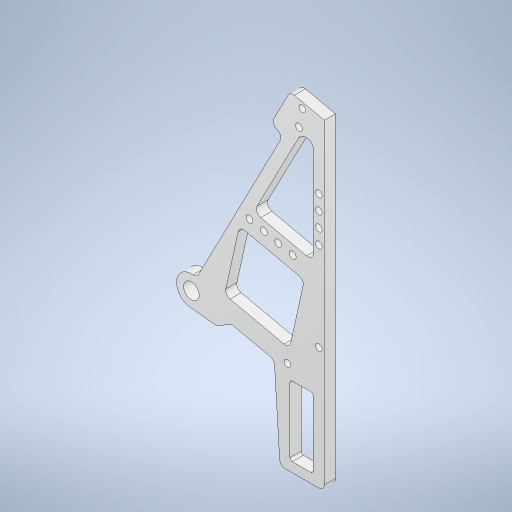
# Autodesk Inventor part: Uprights
Saved by Autodesk Inventor 2023.4 (Build 274418000, 418)
## iProperties
Created: 2024-02-11
Part Number: Uprights
Material: Aluminum 6061
Document SubType Name: Modeling
Designer: Nathan Cai
Density: 2.7 g/cm^3
Appearance: Aluminum - Flat
Mass: 24.6883 g
Surface Area: 68.1147 cm^2
Volume: 9.14381 cm^3
Author: Nathan Cai
Autodesk Inventor part; units mm, degrees
ref_plane "YZ Plane" through (0, 0, 0) normal (1, 0, 0) x (0, 1, 0)
ref_plane "XZ Plane" through (0, 0, 0) normal (0, 1, 0) x (-1, 0, 0)
ref_plane "XY Plane" through (0, 0, 0) normal (0, 0, 1) x (1, 0, 0)
sketch "Sketch1" plane through (0, 0, 0) normal (0, 0, 1) x (1, 0, 0)
  line L0 (0, 0) -> (0, 136.2362)
  line L1 (-14.9636, 12.2907) -> (-42.8613, 18.4755)
  line L2 (-42.8613, 18.4755) -> (-36.5047, 47.1481)
  line L3 (-36.5047, 47.1481) -> (-8.607, 40.9633)
  line L4 (-8.607, 40.9633) -> (-14.9636, 12.2907)
  line L5 (-42.8613, 18.4755) -> (-8.607, 40.9633) construction
  line L6 (-36.5047, 47.1481) -> (-14.9636, 12.2907) construction
  circle A0 centre (-57.15, 12.7) radius 3.3401
  circle A1 centre (-57.15, 12.7) radius 6.35
  line L7 (0, 0) -> (-57.847, 6.3884)
  line L8 (-62.7825, 15.6321) -> (0, 136.2362)
  line L9 (-30.3052, 45.7737) -> (-40.6279, 28.5497)
  line L10 (-14.8065, 42.3377) -> (-12.7302, 22.3649)
  line L11 (-22.5559, 44.0557) -> (-28.9124, 15.3831) construction
  line L12 (0, 104.775) -> (-14.6831, 108.0302)
  line L13 (-40.1014, 8.9204) -> (-21.503, 4.7972)
  line L14 (-21.503, 4.7972) -> (-22.8774, -1.4022)
  line L15 (-22.8774, -1.4022) -> (-41.4758, 2.7209)
  line L16 (-41.4758, 2.7209) -> (-40.1014, 8.9204)
  line L17 (-40.1014, 8.9204) -> (-46.1105, 5.0922)
  line L18 (-21.503, 4.7972) -> (-19.8429, 2.1914)
  line L19 (-8.607, 40.9633) -> (-36.5047, 47.1481)
  line L20 (-36.5047, 47.1481) -> (-35.4225, 52.0296)
  line L21 (-35.4225, 52.0296) -> (-7.5248, 45.8448)
  line L22 (-7.5248, 45.8448) -> (-8.607, 40.9633)
  line L23 (-56.4271, 15.9609) -> (-57.15, 12.7) construction
  line L24 (-57.15, 12.7) -> (-60.4109, 13.4229) construction
  line L25 (-30.8022, 6.8588) -> (-37.6742, -24.1386) construction
  line L26 (-35.0426, 50.076) -> (-8.6948, 44.2349)
  line L27 (-8.6948, 44.2349) -> (-7.664, 48.8845)
  line L28 (-7.664, 48.8845) -> (-34.0118, 54.7256)
  line L29 (-34.0118, 54.7256) -> (-35.0426, 50.076)
  line L30 (-34.5272, 52.4008) -> (-8.1794, 46.5597) construction
  circle A2 centre (-32.2024, 51.8854) radius 1.4732
  circle A3 centre (-26.0029, 50.5111) radius 1.4732
  circle A4 centre (-19.8034, 49.1367) radius 1.4732
  circle A5 centre (-13.6039, 47.7623) radius 1.4732
  circle A6 centre (-10.8735, 96.7513) radius 1.4732
  line L31 (-57.8541, 13.0665) -> (-9.0672, 106.7852)
  line L32 (-35.1857, 56.612) -> (0, 48.8115)
  circle A7 centre (-10.8735, 96.7513) radius 3.175
  line L33 (-4.7625, 49.8673) -> (-4.7625, 105.8308)
  line L34 (-30.3721, 55.5448) -> (-10.5664, 93.5912)
  line L35 (-8.4465, 94.7043) -> (-4.7625, 93.8875)
  circle A8 centre (-15.875, 6.35) radius 1.4224
  line L36 (-9.525, 4.7625) -> (-19.8429, 2.1914)
  line L37 (-9.525, 7.9375) -> (-9.525, 4.7625)
  line L38 (-9.525, 7.9375) -> (0, 7.9375)
  line L39 (0, 13.4938) -> (-4.7625, 13.4937) construction
  line L40 (-4.7625, 13.4937) -> (-4.7625, 24.6063) construction
  line L41 (-4.7625, 24.6063) -> (0, 24.6063) construction
  line L42 (0, 24.6063) -> (0, 13.4938) construction
  line L43 (-4.7625, 19.05) -> (0, 19.05) construction
  circle A9 centre (-2.3812, 19.05) radius 1.4224
  line L44 (-4.7625, 57.15) -> (0, 57.15) construction
  circle A10 centre (-2.3813, 57.15) radius 1.4224
  circle A11 centre (-2.3813, 63.5) radius 1.4224
  circle A12 centre (-2.3813, 69.85) radius 1.4224
  circle A13 centre (-2.3813, 76.2) radius 1.4224
  line L45 (-37.6742, -24.1386) -> (-17.7455, 65.7539) construction
  line L46 (-17.7455, 65.7539) -> (-20.4943, 53.3549) construction
  line L47 (-20.4943, 53.3549) -> (-14.2948, 51.9805) construction
  line L48 (-14.2948, 51.9805) -> (-11.546, 64.3795) construction
  line L49 (-11.546, 64.3795) -> (-17.7455, 65.7539) construction
  line L50 (-17.3945, 52.6677) -> (-14.6458, 65.0667) construction
  line L51 (-19.1199, 59.5544) -> (-12.9204, 58.18) construction
  line L52 (-20.4943, 53.3549) -> (-12.9204, 58.18) construction
  line L53 (-17.7455, 65.7539) -> (-12.9204, 58.18) construction
  circle A14 centre (-16.7073, 55.7675) radius 1.4224
  circle A15 centre (-15.3329, 61.967) radius 1.4224
  line L54 (-17.3945, 52.6677) -> (-15.3329, 61.967) construction
  line L55 (-14.2948, 51.9805) -> (-12.2332, 61.2798)
  line L56 (-18.4327, 62.6542) -> (-20.4943, 53.3549)
  arc A16 (-20.4943, 53.3549) -> (-14.2948, 51.9805) centre (-17.3945, 52.6677) ccw construction
  arc A17 (-12.2332, 61.2798) -> (-18.4327, 62.6542) centre (-15.3329, 61.967) ccw
  line L57 (-22.792, 92.4532) -> (-17.8635, 89.8876)
  arc A18 (0, 104.775) -> (-17.8922, 108.7416) centre (-9.4775, 104.3612) ccw construction
  circle A19 centre (-9.4775, 104.3612) radius 1.4224
  line L58 (-25.9734, 93.2179) -> (-17.8922, 108.7416)
  circle A20 centre (-57.15, 12.7) radius 9.525 construction
  line L59 (-14.7625, 0.7937) -> (-4.7625, 0.7938)
  line L60 (-4.7625, 0.7938) -> (-4.7625, -29.2062)
  line L61 (-4.7625, -29.2062) -> (-14.7625, -29.2062)
  line L62 (-14.7625, -29.2062) -> (-14.7625, 0.7937)
  line L63 (-14.7625, 0.7937) -> (-4.7625, -29.2062) construction
  line L64 (-4.7625, 0.7938) -> (-14.7625, -29.2062) construction
  line L65 (-19.05, -33.3375) -> (0, -33.3375)
  line L66 (0, -33.3375) -> (0, 0)
  line L67 (-21.503, 4.7972) -> (-19.05, -33.3375)
  point P0 (-25.7341, 29.7194)
  point P1 (0, 136.2362)
  point P2 (-22.0272, 2.4326)
  point P3 (-41.0734, 4.536)
  point P4 (-54.945, 18.6549)
  point P5 (0, 48.8115)
  point P6 (-4.7625, 7.9375)
  point P7 (-25.7341, 29.7194)
  point P8 (-16.3637, 57.3173)
  point P9 (-20.4943, 53.3549)
  point P10 (-14.2948, 51.9805)
  point P11 (-7.1364, 106.3571)
  point P12 (-9.7122, 106.9281)
  point P13 (-9.591, 105.7791)
  point P14 (-10.704, 103.6409)
  point P15 (-9.7625, -14.2062)
  dimension "d14" = 29.3687
  dimension "d15" = 28.575
  dimension "d16" = 12.5
  dimension "d17" = 6.6802
  dimension "d19" = 57.15
  dimension "d22" = 12.7
  dimension "d23" = 7.9375
  dimension "d24" = 19.05
  dimension "d26" = 102.5
  dimension "d29" = 6.35
  dimension "d31" = 9.525
  dimension "d34" = 5
  dimension "d35" = 26.9875
  dimension "d38" = 31.75
  dimension "d40" = 26.9875
  dimension "d41" = 4.7625
  dimension "d42" = 2.9464
  dimension "d43" = 2.3813
  dimension "d46" = 6.35
  dimension "d51" = 2.9464
  dimension "d52" = 92.075
  dimension "d53" = 6.35
  dimension "d54" = 6.35
  dimension "d55" = 4.7625
  dimension "d56" = 4.7625
  dimension "d60" = 12.7
  dimension "d61" = 3.175
  dimension "d66" = 2.8448
  dimension "d67" = 15.875
  dimension "d72" = 8.7312
  dimension "d80" = 104.775
  dimension "d81" = 6.35
  dimension "d82" = 7.9375
  dimension "d83" = 3.175
  dimension "d84" = 9.525
  dimension "d85" = 4.7625
  dimension "d86" = 11.1125
  dimension "d87" = 2.8448
  dimension "d88" = 19.05
  dimension "d89" = 2.8448
  dimension "d90" = 38.1
  dimension "d93" = 6.35
  dimension "d98" = 92.075
  dimension "d99" = 12.7
  dimension "d100" = 6.35
  dimension "d101" = 2.8448
  dimension "d102" = 2.8448
  dimension "d104" = 27.5
  dimension "d105" = 5.5563
  dimension "d106" = 19.05
  dimension "d108" = 2.8448
  dimension "d111" = 19.05
  dimension "d112" = 10
  dimension "d113" = 30
  dimension "d114" = 4.7625
  dimension "d115" = 0.7937
  dimension "d116" = 41.275
  dimension "d117" = 19.05
  constraints: 138 end point, 29 point on line, 23 parallel, 21 centre point, 21 midpoint, 14 perpendicular, 12 coincident, 12 point on circle, 10 tangent, 3 horizontal, 3 vertical, 2 collinear, 17 other
  measures "d14" distance of L1.end L2.end
  measures "d15" distance between parallel lines of L4 L2
  measures "d16" angle of L0 L4
  measures "d17" diameter of A0
  measures "d19" distance from line of L0 A0.centre
  measures "d22" diameter of A1
  measures "d23" distance from line of L9.start L11
  measures "d24" distance from line of L9.end L3
  measures "d26" angle of L0 L12
  measures "d29" distance of L13.end L14.end
  measures "d31" distance between parallel lines of L14 L11
  measures "d34" distance of L2.end L20.end
  measures "d35" distance between parallel lines of L11 L23
  measures "d38" distance of L25.start L25.end
  measures "d40" distance between parallel lines of L27 L29
  measures "d41" distance between parallel lines of L26 L28
  measures "d42" diameter of A2
  measures "d43" distance from line of L29 A2.centre
  measures "d46" distance of A2.centre A3.centre
  measures "d51" diameter of A6
  measures "d52" distance from line of L13 A6.centre
  measures "d53" distance between parallel lines of L32 L26
  measures "d54" diameter of A7
  measures "d55" distance between parallel lines of L0 L33
  measures "d56" distance between parallel lines of L31 L34
  measures "d60" vertical distance of A0.centre L0.start
  measures "d61" distance between parallel lines of L3 L26
  measures "d66" diameter of A8
  measures "d67" distance from line of L0 A8.centre
  measures "d72" distance between parallel lines of L1 L13
  measures "d80" distance of L0.start point (0, 104.775)
  measures "d81" vertical distance of L0.start A8.centre
  measures "d82" distance from line of L0.start L38
  measures "d83" vertical distance of point (-4.763, 7.937) L36.start
  measures "d84" distance between parallel lines of L0 L37
  measures "d85" distance of L40.end L41.end
  measures "d86" distance between parallel lines of L39 L41
  measures "d87" diameter of A9
  measures "d88" distance from line of L66.end L43
  measures "d89" diameter of A10
  measures "d90" distance between parallel lines of L43 L44
  measures "d93" distance of A10.centre A11.centre
  measures "d98" distance of L25.end L45.end
  measures "d99" distance of L45.end L46.end
  measures "d100" distance of L47.end L46.end
  measures "d101" diameter of A14
  measures "d102" diameter of A15
  measures "d104" angle of L0 L8
  measures "d105" distance between parallel lines of L8 L31
  measures "d106" distance from line of L31.end L57
  measures "d108" diameter of A19
  measures "d111" diameter of A20
  measures "d112" distance of L60.end L61.end
  measures "d113" distance of L59.end L60.end
  measures "d114" distance between parallel lines of L0 L60
  measures "d115" distance from line of L0.start L59
  measures "d116" distance between parallel lines of L38 L65
  measures "d117" distance of L65.start L65.end
extrude "Extrusion1" add sketch "Sketch1" along normal blind 4.7625 contours L7 L60 L59 L36 L37 L38 L0 | L66 L65 L67 L7 L59 L62 L61 L60 | L38 L37 L36 L18 L13 L17 L7 A1 L31 L32 L0 | L32 L33 L12 L0 | L7 L67 L18 | L33 L35 A7 L31 A19 L12 | L12 L31 A19 A7 L57 L8 | A7 L31 | L32 L31 A7 L34 | A1 | A7 L31 | L3 L20 L21 L29 L26 L27 L22 | L27 L26 L29 L21 A2 A3 A4 A5 | L21 A5 A4 A3 A2 L29 L28 L27
fillet "Fillet1" radius 2.3813 18 edges at (-42.8613, 18.4755, 2.3813) (-14.9636, 12.2907, 2.3813) (-54.945, 18.6549, 2.3813) (-21.503, 4.7972, 2.3813) (-40.1014, 8.9204, 2.3813) (-46.1105, 5.0922, 2.3813) (-10.5664, 93.5912, 2.3813) (-8.4465, 94.7043, 2.3813) (-4.7625, 93.8875, 2.3813) (-30.3721, 55.5448, 2.3813) (-4.7625, 49.8673, 2.3813) (-36.5047, 47.1481, 2.3813) (-8.607, 40.9633, 2.3813) (-17.8635, 89.8876, 2.3813) (-22.792, 92.4532, 2.3813) (-14.6831, 108.0302, 2.3813) (-19.05, -33.3375, 2.3813) (0, -33.3375, 2.3813)
fillet "Fillet6" radius 1 4 edges at (-4.7625, 0.7938, 2.3813) (-14.7625, 0.7937, 2.3813) (-14.7625, -29.2062, 2.3813) (-4.7625, -29.2062, 2.3813)
equation "\"d56\" = d55"
body "Solid1"
